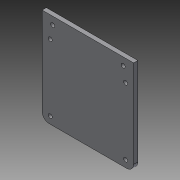
# Autodesk Inventor part: electronics_pouch
Saved by Autodesk Inventor 2014 SP1 (Build 180222100, 222)
## iProperties
Created: 2014-11-09
Part Number: electronics_pouch
Material: Generic
Document SubType Name: Modeling
Designer: rawrdong
Density: 1 g/cm^3
Appearance: Default
Author: rawrdong
Autodesk Inventor part; units mm, degrees
ref_plane "YZ Plane" through (0, 0, 0) normal (1, 0, 0) x (0, 1, 0)
ref_plane "XZ Plane" through (0, 0, 0) normal (0, 1, 0) x (-1, 0, 0)
ref_plane "XY Plane" through (0, 0, 0) normal (0, 0, 1) x (1, 0, 0)
sketch "Sketch1" plane through (0, 0, 0) normal (0, 1, 0) x (-1, 0, 0)
  line L0 (0, 0) -> (65, 0)
  line L1 (65, 0) -> (65, -67.32)
  line L2 (65, -67.32) -> (0, -67.32)
  line L3 (0, -67.32) -> (0, 0)
  circle A0 centre (7.5, -5.4) radius 1.425
  circle A1 centre (57.5, -5.4) radius 1.425
  line L4 (32.5, 0) -> (32.5, -67.32) construction
  circle A2 centre (5.765, -15) radius 1.425
  circle A3 centre (5.765, -62.32) radius 1.425
  circle A4 centre (59.235, -15) radius 1.425
  circle A5 centre (59.235, -62.32) radius 1.425
  line L5 (5.765, -15) -> (59.235, -15) construction
  line L6 (59.235, -15) -> (59.235, -62.32) construction
  line L7 (59.235, -62.32) -> (5.765, -62.32) construction
  line L8 (5.765, -62.32) -> (5.765, -15) construction
  dimension "d0" = 65
  dimension "d1" = 2.85
  dimension "d2" = 50
  dimension "d3" = 5.4
  dimension "d4" = 53.47
  dimension "d5" = 47.32
  dimension "d6" = 15
  dimension "d7" = 5
  constraints: 18 end point, 6 centre point, 5 equal radius, 4 parallel, 2 coincident, 2 horizontal, 2 midpoint, 2 perpendicular, 1 horizontal alignment, 1 symmetric about line, 1 other
  measures "d0" distance of L0.start L0.end
  measures "d1" diameter of A0
  measures "d2" distance of A1.centre A0.centre
  measures "d3" distance from line of L0 A0.centre
  measures "d4" distance of L6.end L7.end
  measures "d5" distance of L5.end L6.end
  measures "d6" distance between parallel lines of L0 L5
  measures "d7" distance between parallel lines of L7 L2
extrude "Extrusion1" add sketch "Sketch1" along normal blind 3
fillet "Fillet1" radius 5 2 edges at (0, 1.5, -67.32) (-65, 1.5, -67.32)
body "Solid1"
